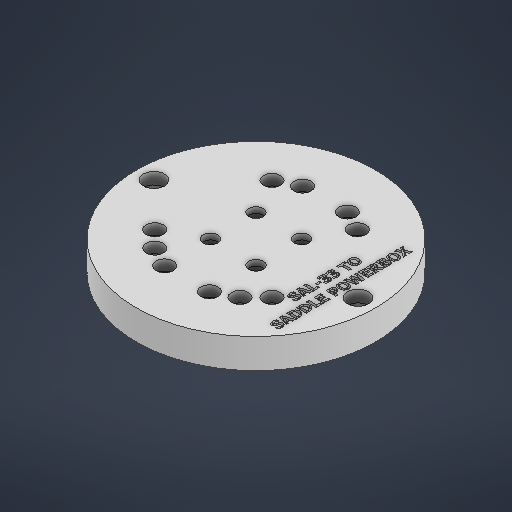
# Autodesk Inventor part: SAL-33 to Saddle Powerbox Adapter
Saved by Autodesk Inventor 2026.2 (Build 302298010, 298A)
## iProperties
Created: 2026-05-21
Part Number: SAL-33 to Saddle Powerbox Adapter
Material: Generic
Document SubType Name: Modeling
Designer: incep
Density: 1 g/cm^3
Appearance: Default
Author: incep
## iProperties of the stored document SAL-33 to Saddle Powerbox Adapter_3DPrint.ipt
Created: 2026-05-21
Part Number: SAL-33 to Saddle Powerbox Adapter_3DPrint
Material: Generic
Document SubType Name: Modeling
Designer: incep
Density: 1 g/cm^3
Appearance: Default
Author: incep
Autodesk Inventor part; units mm, degrees
ref_plane "YZ Plane" through (0, 0, 0) normal (1, 0, 0) x (0, 1, 0)
ref_plane "XZ Plane" through (0, 0, 0) normal (0, 1, 0) x (-1, 0, 0)
ref_plane "XY Plane" through (0, 0, 0) normal (0, 0, 1) x (1, 0, 0)
sketch "Sketch1" plane through (0, 0, 0) normal (0, 1, 0) x (-1, 0, 0)
  circle A0 centre (0, 0) radius 44.5
  circle A1 centre (0, 0) radius 22.75
  circle A2 centre (0, 0) radius 27 construction
  circle A3 centre (0, 27) radius 1.925 construction
  circle A4 centre (-8.3435, 25.6785) radius 1.925
  circle A5 centre (-15.8702, 21.8435) radius 1.925
  circle A6 centre (-21.8435, 15.8702) radius 1.925
  circle A7 centre (-25.6785, 8.3435) radius 1.925 construction
  circle A8 centre (-27, 0) radius 1.925 construction
  circle A9 centre (-25.6785, -8.3435) radius 1.925 construction
  circle A10 centre (-21.8435, -15.8702) radius 1.925 construction
  circle A11 centre (-15.8702, -21.8435) radius 1.925
  circle A12 centre (-8.3435, -25.6785) radius 1.925
  circle A13 centre (0, -27) radius 1.925 construction
  circle A14 centre (8.3435, -25.6785) radius 1.925
  circle A15 centre (15.8702, -21.8435) radius 1.925
  circle A16 centre (21.8435, -15.8702) radius 1.925 construction
  circle A17 centre (25.6785, -8.3435) radius 1.925 construction
  circle A18 centre (27, 0) radius 1.925 construction
  circle A19 centre (25.6785, 8.3435) radius 1.925 construction
  circle A20 centre (21.8435, 15.8702) radius 1.925
  circle A21 centre (15.8702, 21.8435) radius 1.925
  circle A22 centre (8.3435, 25.6785) radius 1.925
  dimension "d2" = 54
  dimension "d0" = 89
  dimension "d1" = 45.5
  dimension "d3" = 3.85
  dimension "d6" = 360
  constraints: 22 centre point, 3 coincident, 1 vertical alignment, 43 other
  measures "d0" diameter of A0
  measures "d1" diameter of A1
  measures "d3" diameter of A3
extrude "Extrusion1" add sketch "Sketch1" along normal blind 3
sketch "Sketch2" plane through (0, 3, 0) normal (0, 1, 0) x (1, 0, 0)
  circle A0 centre (0, 0) radius 22.75 projected
  circle A1 centre (0, 0) radius 44.5 projected
  circle A2 centre (-8.3435, -25.6785) radius 1.925 projected
  circle A3 centre (-15.8702, -21.8435) radius 1.925 projected
  circle A4 centre (-21.8435, -15.8702) radius 1.925 projected
  circle A5 centre (-15.8702, 21.8435) radius 1.925 projected
  circle A6 centre (-8.3435, 25.6785) radius 1.925 projected
  circle A7 centre (8.3435, 25.6785) radius 1.925 projected
  circle A8 centre (15.8702, 21.8435) radius 1.925 projected
  circle A9 centre (21.8435, -15.8702) radius 1.925 projected
  circle A10 centre (15.8702, -21.8435) radius 1.925 projected
  circle A11 centre (8.3435, -25.6785) radius 1.925 projected
  circle A12 centre (0, 0) radius 22.75 projected
extrude "Extrusion2" add sketch "Sketch2" along normal blind 8 contours A0 | A1
sketch "Sketch3" plane through (0, 11, 0) normal (0, 1, 0) x (1, 0, 0)
  circle A0 centre (0, 0) radius 44.5 projected
  circle A1 centre (0, 0) radius 44.5 projected
  circle A2 centre (8.3435, -25.6785) radius 1.925 projected
  circle A3 centre (15.8702, -21.8435) radius 1.925 projected
  circle A4 centre (21.8435, -15.8702) radius 1.925 projected
  circle A5 centre (15.8702, 21.8435) radius 1.925 projected
  circle A6 centre (8.3435, 25.6785) radius 1.925 projected
  circle A7 centre (-8.3435, 25.6785) radius 1.925 projected
  circle A8 centre (-15.8702, 21.8435) radius 1.925 projected
  circle A9 centre (-21.8435, -15.8702) radius 1.925 projected
  circle A10 centre (-15.8702, -21.8435) radius 1.925 projected
  circle A11 centre (-8.3435, -25.6785) radius 1.925 projected
  circle A12 centre (-8.3435, -25.6785) radius 3.2
  circle A13 centre (-21.8435, -15.8702) radius 3.2
  circle A14 centre (-15.8702, -21.8435) radius 3.2
  circle A15 centre (8.3435, -25.6785) radius 3.2
  circle A16 centre (15.8702, -21.8435) radius 3.2
  circle A17 centre (21.8435, -15.8702) radius 3.2
  circle A18 centre (15.8702, 21.8435) radius 3.2
  circle A19 centre (8.3435, 25.6785) radius 3.2
  circle A20 centre (-8.3435, 25.6785) radius 3.2
  circle A21 centre (-15.8702, 21.8435) radius 3.2
  dimension "d12" = 6.4
  dimension "d13" = 6.4
  dimension "d14" = 6.4
  dimension "d15" = 6.4
  dimension "d16" = 6.4
  dimension "d17" = 6.4
  dimension "d18" = 6.4
  dimension "d19" = 6.4
  dimension "d20" = 6.4
  dimension "d21" = 6.4
  constraints: 10 centre point, 10 coincident
  measures "d12" diameter of A12
  measures "d13" diameter of A13
  measures "d14" diameter of A14
  measures "d15" diameter of A15
  measures "d16" diameter of A16
  measures "d17" diameter of A17
  measures "d18" diameter of A18
  measures "d19" diameter of A19
  measures "d20" diameter of A20
  measures "d21" diameter of A21
extrude "Extrusion3" cut sketch "Sketch3" against normal blind 4 contours A2 | A3 | A4 | A5 | A6 | A7 | A8 | A9 | A10 | A11 | A12 | A13 | A14 | A15 | A16 | A17 | A18 | A19 | A20 | A21
sketch "Sketch4" plane through (0, 11, 0) normal (0, 1, 0) x (1, 0, 0)
  circle A0 centre (-38, 0) radius 3.925
  circle A1 centre (38, 0) radius 3.925
  line L0 (-38, 0) -> (38, 0) construction
  circle A2 centre (-38, 0) radius 2.25
  circle A3 centre (38, 0) radius 2.25
  point P0 (0, 0)
  point P1 (0, 0)
  dimension "d24" = 7.85
  dimension "d25" = 76
  dimension "d26" = 4.5
  constraints: 4 centre point, 3 coincident, 2 end point, 2 equal radius, 2 horizontal alignment, 1 horizontal, 1 midpoint
  measures "d24" diameter of A0
  measures "d25" distance of L0.end L0.start
  measures "d26" diameter of A2
extrude "Extrusion4" cut sketch "Sketch4" against normal blind 4.36 contours A0 | A1 | A2 | A3
extrude "Extrusion5" cut sketch "Sketch4" against normal up to surface (11 mm away) contours A2 | A3
sketch "Sketch5" plane through (0, 11, 0) normal (0, 1, 0) x (1, 0, 0)
  line L0 (-8.5, -8.5) -> (8.5, -8.5) construction
  line L1 (8.5, -8.5) -> (8.5, 8.5) construction
  line L2 (8.5, 8.5) -> (-8.5, 8.5) construction
  line L3 (-8.5, 8.5) -> (-8.5, -8.5) construction
  circle A0 centre (-8.5, -8.5) radius 2.7
  circle A1 centre (-8.5, 8.5) radius 2.7
  circle A2 centre (8.5, 8.5) radius 2.7
  circle A3 centre (8.5, -8.5) radius 2.7
  circle A4 centre (0, 0) radius 12.0208 construction
  point P0 (-8.5, 0)
  point P1 (0, 8.5)
  dimension "d40" = 24.0416
  dimension "d31" = 5.4
  dimension "d37" = 17
  constraints: 8 end point, 5 coincident, 4 centre point, 3 equal radius, 2 midpoint, 2 parallel, 2 perpendicular, 1 horizontal, 1 horizontal alignment, 1 vertical alignment, 3 other
  measures "d31" diameter of A0
  measures "d37" distance of L0.start L0.end
extrude "Extrusion6" cut sketch "Sketch5" against normal up to surface (8 mm away)
sketch "Sketch6" plane through (0, 3, 0) normal (0, -1, 0) x (1, 0, 0)
  circle A0 centre (8.5, -8.5) radius 2.7 projected
  circle A1 centre (-8.5, 8.5) radius 2.7 projected
  circle A2 centre (-8.5, -8.5) radius 2.7 projected
  circle A3 centre (8.5, 8.5) radius 2.7 projected
  circle A4 centre (0, 0) radius 22.75 projected
  circle A5 centre (-8.5, 8.5) radius 3.2
  circle A6 centre (8.5, 8.5) radius 3.2
  circle A7 centre (-8.5, -8.5) radius 3.2
  circle A8 centre (8.5, -8.5) radius 3.2
  dimension "d34" = 6.4
  constraints: 4 centre point, 4 coincident, 3 equal radius
  measures "d34" diameter of A5
extrude "Extrusion7" cut sketch "Sketch6" against normal blind 5.8 contours A0 | A1 | A2 | A3 | A5 | A6 | A7 | A8
sketch "Sketch7" plane through (0, 11, 0) normal (0, 1, 0) x (1, 0, 0)
  line L0 (23.7791, -32.5352) -> (23.7791, 32.5352) construction
  line L1 (23.7791, 32.5352) -> (26.5195, 32.5352) construction
  line L2 (26.5195, 32.5352) -> (26.5195, -32.5352) construction
  line L3 (26.5195, -32.5352) -> (23.7791, -32.5352) construction
  spline S0 degree 2 poles (27.4734, -11.4216) (27.4734, -11.8308) (27.3149, -12.4474) (27.1997, -12.7126) knots 0 0 0 1 2 2 2
  line L4 (27.1997, -12.7126) -> (26.3525, -12.7126)
  line L5 (26.3525, -12.7126) -> (26.3525, -12.6319)
  spline S1 degree 2 poles (26.3525, -12.6319) (26.5801, -12.3639) (26.825, -11.7213) (26.825, -11.4187) knots 0 0 0 1 2 2 2
  spline S2 degree 2 poles (26.825, -11.4187) (26.825, -11.3409) (26.7905, -11.0902) (26.7559, -11.0152) knots 0 0 0 1 2 2 2
  spline S3 degree 2 poles (26.7559, -11.0152) (26.7155, -10.923) (26.5686, -10.7934) (26.4504, -10.7934) knots 0 0 0 1 2 2 2
  spline S4 degree 2 poles (26.4504, -10.7934) (26.315, -10.7934) (26.1479, -11.0037) (26.1104, -11.1478) knots 0 0 0 1 2 2 2
  spline S5 degree 2 poles (26.1104, -11.1478) (26.0614, -11.3293) (25.9778, -11.7414) (25.9144, -11.923) knots 0 0 0 1 2 2 2
  spline S6 degree 2 poles (25.9144, -11.923) (25.7704, -12.3351) (25.2776, -12.6924) (24.9087, -12.6924) knots 0 0 0 1 2 2 2
  spline S7 degree 2 poles (24.9087, -12.6924) (24.4102, -12.6924) (23.7906, -11.8481) (23.7906, -11.2141) knots 0 0 0 1 2 2 2
  spline S8 degree 2 poles (23.7906, -11.2141) (23.7906, -10.8971) (23.9203, -10.2689) (24.0298, -10.0211) knots 0 0 0 1 2 2 2
  line L6 (24.0298, -10.0211) -> (24.8424, -10.0211)
  line L7 (24.8424, -10.0211) -> (24.8424, -10.0989)
  spline S9 degree 2 poles (24.8424, -10.0989) (24.6724, -10.2977) (24.439, -10.8683) (24.439, -11.168) knots 0 0 0 1 2 2 2
  spline S10 degree 2 poles (24.439, -11.168) (24.439, -11.2861) (24.4736, -11.4705) (24.5197, -11.5743) knots 0 0 0 1 2 2 2
  spline S11 degree 2 poles (24.5197, -11.5743) (24.5572, -11.6579) (24.707, -11.7789) (24.7992, -11.7789) knots 0 0 0 1 2 2 2
  spline S12 degree 2 poles (24.7992, -11.7789) (24.9375, -11.7789) (25.096, -11.5858) (25.1594, -11.3092) knots 0 0 0 1 2 2 2
  spline S13 degree 2 poles (25.1594, -11.3092) (25.1998, -11.1305) (25.2776, -10.7991) (25.3439, -10.6089) knots 0 0 0 1 2 2 2
  spline S14 degree 2 poles (25.3439, -10.6089) (25.4793, -10.2401) (25.9288, -9.8799) (26.2977, -9.8799) knots 0 0 0 1 2 2 2
  spline S15 degree 2 poles (26.2977, -9.8799) (26.8279, -9.8799) (27.4734, -10.7127) (27.4734, -11.4216) knots 0 0 0 1 2 2 2
  line L8 (27.41, -9.8049) -> (23.854, -8.6033)
  line L9 (23.854, -8.6033) -> (23.854, -7.6293)
  line L10 (23.854, -7.6293) -> (27.41, -6.4276)
  line L11 (27.41, -6.4276) -> (27.41, -7.3469)
  line L12 (27.41, -7.3469) -> (26.6838, -7.5687)
  line L13 (26.6838, -7.5687) -> (26.6838, -8.6868)
  line L14 (26.6838, -8.6868) -> (27.41, -8.9116)
  line L15 (27.41, -8.9116) -> (27.41, -9.8049)
  line L16 (26.0383, -7.7647) -> (24.8626, -8.1278)
  line L17 (24.8626, -8.1278) -> (26.0383, -8.4938)
  line L18 (26.0383, -8.4938) -> (26.0383, -7.7647)
  line L19 (27.41, -3.7015) -> (27.41, -6.0732)
  line L20 (27.41, -6.0732) -> (23.854, -6.0732)
  line L21 (23.854, -6.0732) -> (23.854, -5.1798)
  line L22 (23.854, -5.1798) -> (26.7328, -5.1798)
  line L23 (26.7328, -5.1798) -> (26.7328, -3.7015)
  line L24 (26.7328, -3.7015) -> (27.41, -3.7015)
  line L25 (26.1709, -1.7996) -> (26.1709, -3.3817)
  line L26 (26.1709, -3.3817) -> (25.5081, -3.3817)
  line L27 (25.5081, -3.3817) -> (25.5081, -1.7996)
  line L28 (25.5081, -1.7996) -> (26.1709, -1.7996)
  spline S16 degree 2 poles (26.3323, 1.3501) (26.5945, 1.3501) (27.0239, 1.157) (27.1737, 0.9697) knots 0 0 0 1 2 2 2
  spline S17 degree 2 poles (27.1737, 0.9697) (27.3236, 0.7824) (27.485, 0.2723) (27.485, -0.0937) knots 0 0 0 1 2 2 2
  spline S18 degree 2 poles (27.485, -0.0937) (27.485, -0.5086) (27.3466, -1.1022) (27.2602, -1.2896) knots 0 0 0 1 2 2 2
  line L29 (27.2602, -1.2896) -> (26.4879, -1.2896)
  line L30 (26.4879, -1.2896) -> (26.4879, -1.2031)
  spline S19 degree 2 poles (26.4879, -1.2031) (26.6118, -1.0071) (26.7962, -0.4798) (26.7962, -0.2608) knots 0 0 0 1 2 2 2
  spline S20 degree 2 poles (26.7962, -0.2608) (26.7962, -0.1311) (26.7501, 0.1715) (26.6752, 0.2752) knots 0 0 0 1 2 2 2
  spline S21 degree 2 poles (26.6752, 0.2752) (26.6147, 0.3559) (26.4389, 0.4539) (26.2804, 0.4539) knots 0 0 0 1 2 2 2
  spline S22 degree 2 poles (26.2804, 0.4539) (26.1219, 0.4539) (25.9519, 0.3155) (25.9116, 0.2003) knots 0 0 0 1 2 2 2
  spline S23 degree 2 poles (25.9116, 0.2003) (25.8712, 0.085) (25.8626, -0.2349) (25.8626, -0.3588) knots 0 0 0 1 2 2 2
  line L31 (25.8626, -0.3588) -> (25.8626, -0.5115)
  line L32 (25.8626, -0.5115) -> (25.2372, -0.5115)
  line L33 (25.2372, -0.5115) -> (25.2372, -0.3703)
  spline S24 degree 2 poles (25.2372, -0.3703) (25.2372, -0.2089) (25.2084, 0.0648) (25.1652, 0.1599) knots 0 0 0 1 2 2 2
  spline S25 degree 2 poles (25.1652, 0.1599) (25.1191, 0.255) (24.9577, 0.3617) (24.8194, 0.3617) knots 0 0 0 1 2 2 2
  spline S26 degree 2 poles (24.8194, 0.3617) (24.7099, 0.3617) (24.5745, 0.2608) (24.537, 0.1888) knots 0 0 0 1 2 2 2
  spline S27 degree 2 poles (24.537, 0.1888) (24.4938, 0.1023) (24.4649, -0.1282) (24.4649, -0.2089) knots 0 0 0 1 2 2 2
  spline S28 degree 2 poles (24.4649, -0.2089) (24.4649, -0.3386) (24.5255, -0.6124) (24.5745, -0.7392) knots 0 0 0 1 2 2 2
  spline S29 degree 2 poles (24.5745, -0.7392) (24.6119, -0.84) (24.7329, -1.059) (24.7646, -1.1109) knots 0 0 0 1 2 2 2
  line L34 (24.7646, -1.1109) -> (24.7646, -1.1858)
  line L35 (24.7646, -1.1858) -> (24.0039, -1.1858)
  spline S30 degree 2 poles (24.0039, -1.1858) (23.9261, -1.0014) (23.7791, -0.3789) (23.7791, -0.0533) knots 0 0 0 1 2 2 2
  spline S31 degree 2 poles (23.7791, -0.0533) (23.7791, 0.2637) (23.8886, 0.7305) (23.9952, 0.8948) knots 0 0 0 1 2 2 2
  spline S32 degree 2 poles (23.9952, 0.8948) (24.1076, 1.0763) (24.4534, 1.2579) (24.6695, 1.2579) knots 0 0 0 1 2 2 2
  spline S33 degree 2 poles (24.6695, 1.2579) (24.975, 1.2579) (25.4303, 0.9063) (25.4966, 0.6181) knots 0 0 0 1 2 2 2
  line L36 (25.4966, 0.6181) -> (25.5312, 0.6181)
  spline S34 degree 2 poles (25.5312, 0.6181) (25.5485, 0.7449) (25.6407, 0.987) (25.7444, 1.1022) knots 0 0 0 1 2 2 2
  spline S35 degree 2 poles (25.7444, 1.1022) (25.8366, 1.2089) (26.1306, 1.3501) (26.3323, 1.3501) knots 0 0 0 1 2 2 2
  spline S36 degree 2 poles (26.3323, 4.4652) (26.5945, 4.4652) (27.0239, 4.2721) (27.1737, 4.0848) knots 0 0 0 1 2 2 2
  spline S37 degree 2 poles (27.1737, 4.0848) (27.3236, 3.8975) (27.485, 3.3874) (27.485, 3.0214) knots 0 0 0 1 2 2 2
  spline S38 degree 2 poles (27.485, 3.0214) (27.485, 2.6065) (27.3466, 2.0129) (27.2602, 1.8255) knots 0 0 0 1 2 2 2
  line L37 (27.2602, 1.8255) -> (26.4879, 1.8255)
  line L38 (26.4879, 1.8255) -> (26.4879, 1.912)
  spline S39 degree 2 poles (26.4879, 1.912) (26.6118, 2.108) (26.7962, 2.6353) (26.7962, 2.8543) knots 0 0 0 1 2 2 2
  spline S40 degree 2 poles (26.7962, 2.8543) (26.7962, 2.984) (26.7501, 3.2866) (26.6752, 3.3903) knots 0 0 0 1 2 2 2
  spline S41 degree 2 poles (26.6752, 3.3903) (26.6147, 3.471) (26.4389, 3.569) (26.2804, 3.569) knots 0 0 0 1 2 2 2
  spline S42 degree 2 poles (26.2804, 3.569) (26.1219, 3.569) (25.9519, 3.4306) (25.9116, 3.3154) knots 0 0 0 1 2 2 2
  spline S43 degree 2 poles (25.9116, 3.3154) (25.8712, 3.2001) (25.8626, 2.8802) (25.8626, 2.7563) knots 0 0 0 1 2 2 2
  line L39 (25.8626, 2.7563) -> (25.8626, 2.6036)
  line L40 (25.8626, 2.6036) -> (25.2372, 2.6036)
  line L41 (25.2372, 2.6036) -> (25.2372, 2.7448)
  spline S44 degree 2 poles (25.2372, 2.7448) (25.2372, 2.9062) (25.2084, 3.1799) (25.1652, 3.275) knots 0 0 0 1 2 2 2
  spline S45 degree 2 poles (25.1652, 3.275) (25.1191, 3.3701) (24.9577, 3.4768) (24.8194, 3.4768) knots 0 0 0 1 2 2 2
  spline S46 degree 2 poles (24.8194, 3.4768) (24.7099, 3.4768) (24.5745, 3.3759) (24.537, 3.3039) knots 0 0 0 1 2 2 2
  spline S47 degree 2 poles (24.537, 3.3039) (24.4938, 3.2174) (24.4649, 2.9869) (24.4649, 2.9062) knots 0 0 0 1 2 2 2
  spline S48 degree 2 poles (24.4649, 2.9062) (24.4649, 2.7765) (24.5255, 2.5027) (24.5745, 2.3759) knots 0 0 0 1 2 2 2
  spline S49 degree 2 poles (24.5745, 2.3759) (24.6119, 2.2751) (24.7329, 2.0561) (24.7646, 2.0042) knots 0 0 0 1 2 2 2
  line L42 (24.7646, 2.0042) -> (24.7646, 1.9293)
  line L43 (24.7646, 1.9293) -> (24.0039, 1.9293)
  spline S50 degree 2 poles (24.0039, 1.9293) (23.9261, 2.1137) (23.7791, 2.7362) (23.7791, 3.0618) knots 0 0 0 1 2 2 2
  spline S51 degree 2 poles (23.7791, 3.0618) (23.7791, 3.3788) (23.8886, 3.8456) (23.9952, 4.0099) knots 0 0 0 1 2 2 2
  spline S52 degree 2 poles (23.9952, 4.0099) (24.1076, 4.1914) (24.4534, 4.373) (24.6695, 4.373) knots 0 0 0 1 2 2 2
  spline S53 degree 2 poles (24.6695, 4.373) (24.975, 4.373) (25.4303, 4.0214) (25.4966, 3.7332) knots 0 0 0 1 2 2 2
  line L44 (25.4966, 3.7332) -> (25.5312, 3.7332)
  spline S54 degree 2 poles (25.5312, 3.7332) (25.5485, 3.86) (25.6407, 4.1021) (25.7444, 4.2173) knots 0 0 0 1 2 2 2
  spline S55 degree 2 poles (25.7444, 4.2173) (25.8366, 4.324) (26.1306, 4.4652) (26.3323, 4.4652) knots 0 0 0 1 2 2 2
  line L45 (27.41, 7.1797) -> (24.5312, 7.1797)
  line L46 (24.5312, 7.1797) -> (24.5312, 6.1279)
  line L47 (24.5312, 6.1279) -> (23.854, 6.1279)
  line L48 (23.854, 6.1279) -> (23.854, 9.1249)
  line L49 (23.854, 9.1249) -> (24.5312, 9.1249)
  line L50 (24.5312, 9.1249) -> (24.5312, 8.073)
  line L51 (24.5312, 8.073) -> (27.41, 8.073)
  line L52 (27.41, 8.073) -> (27.41, 7.1797)
  spline S56 degree 2 poles (25.632, 12.727) (26.4965, 12.727) (27.485, 11.8048) (27.485, 11.0037) knots 0 0 0 1 2 2 2
  spline S57 degree 2 poles (27.485, 11.0037) (27.485, 10.1997) (26.485, 9.2834) (25.632, 9.2834) knots 0 0 0 1 2 2 2
  spline S58 degree 2 poles (25.632, 9.2834) (24.7762, 9.2834) (23.7791, 10.1997) (23.7791, 11.0037) knots 0 0 0 1 2 2 2
  spline S59 degree 2 poles (23.7791, 11.0037) (23.7791, 11.8048) (24.7704, 12.727) (25.632, 12.727) knots 0 0 0 1 2 2 2
  spline S60 degree 2 poles (25.632, 11.8048) (25.3122, 11.8048) (24.8655, 11.6751) (24.7243, 11.5628) knots 0 0 0 1 2 2 2
  spline S61 degree 2 poles (24.7243, 11.5628) (24.5773, 11.4504) (24.4505, 11.1622) (24.4505, 11.0066) knots 0 0 0 1 2 2 2
  spline S62 degree 2 poles (24.4505, 11.0066) (24.4505, 10.8423) (24.5687, 10.5743) (24.7185, 10.4504) knots 0 0 0 1 2 2 2
  spline S63 degree 2 poles (24.7185, 10.4504) (24.8569, 10.3409) (25.315, 10.2055) (25.632, 10.2055) knots 0 0 0 1 2 2 2
  spline S64 degree 2 poles (25.632, 10.2055) (25.9605, 10.2055) (26.3928, 10.3352) (26.5398, 10.4476) knots 0 0 0 1 2 2 2
  spline S65 degree 2 poles (26.5398, 10.4476) (26.6867, 10.5599) (26.8135, 10.851) (26.8135, 11.0066) knots 0 0 0 1 2 2 2
  spline S66 degree 2 poles (26.8135, 11.0066) (26.8135, 11.1651) (26.6781, 11.459) (26.534, 11.5656) knots 0 0 0 1 2 2 2
  spline S67 degree 2 poles (26.534, 11.5656) (26.3784, 11.6809) (25.9663, 11.8048) (25.632, 11.8048) knots 0 0 0 1 2 2 2
  spline S68 degree 2 poles (33.3283, -23.6241) (33.3283, -24.0333) (33.1698, -24.6499) (33.0545, -24.9151) knots 0 0 0 1 2 2 2
  line L53 (33.0545, -24.9151) -> (32.2073, -24.9151)
  line L54 (32.2073, -24.9151) -> (32.2073, -24.8344)
  spline S69 degree 2 poles (32.2073, -24.8344) (32.435, -24.5664) (32.6799, -23.9238) (32.6799, -23.6212) knots 0 0 0 1 2 2 2
  spline S70 degree 2 poles (32.6799, -23.6212) (32.6799, -23.5434) (32.6453, -23.2927) (32.6107, -23.2177) knots 0 0 0 1 2 2 2
  spline S71 degree 2 poles (32.6107, -23.2177) (32.5704, -23.1255) (32.4234, -22.9958) (32.3053, -22.9958) knots 0 0 0 1 2 2 2
  spline S72 degree 2 poles (32.3053, -22.9958) (32.1699, -22.9958) (32.0027, -23.2062) (31.9653, -23.3503) knots 0 0 0 1 2 2 2
  spline S73 degree 2 poles (31.9653, -23.3503) (31.9163, -23.5318) (31.8327, -23.9439) (31.7693, -24.1255) knots 0 0 0 1 2 2 2
  spline S74 degree 2 poles (31.7693, -24.1255) (31.6252, -24.5376) (31.1324, -24.8949) (30.7636, -24.8949) knots 0 0 0 1 2 2 2
  spline S75 degree 2 poles (30.7636, -24.8949) (30.2651, -24.8949) (29.6455, -24.0505) (29.6455, -23.4166) knots 0 0 0 1 2 2 2
  spline S76 degree 2 poles (29.6455, -23.4166) (29.6455, -23.0996) (29.7752, -22.4714) (29.8847, -22.2236) knots 0 0 0 1 2 2 2
  line L55 (29.8847, -22.2236) -> (30.6973, -22.2236)
  line L56 (30.6973, -22.2236) -> (30.6973, -22.3014)
  spline S77 degree 2 poles (30.6973, -22.3014) (30.5273, -22.5002) (30.2939, -23.0708) (30.2939, -23.3705) knots 0 0 0 1 2 2 2
  spline S78 degree 2 poles (30.2939, -23.3705) (30.2939, -23.4886) (30.3285, -23.673) (30.3746, -23.7768) knots 0 0 0 1 2 2 2
  spline S79 degree 2 poles (30.3746, -23.7768) (30.412, -23.8604) (30.5619, -23.9814) (30.6541, -23.9814) knots 0 0 0 1 2 2 2
  spline S80 degree 2 poles (30.6541, -23.9814) (30.7924, -23.9814) (30.9509, -23.7883) (31.0143, -23.5117) knots 0 0 0 1 2 2 2
  spline S81 degree 2 poles (31.0143, -23.5117) (31.0546, -23.333) (31.1324, -23.0016) (31.1987, -22.8114) knots 0 0 0 1 2 2 2
  spline S82 degree 2 poles (31.1987, -22.8114) (31.3342, -22.4426) (31.7837, -22.0824) (32.1526, -22.0824) knots 0 0 0 1 2 2 2
  spline S83 degree 2 poles (32.1526, -22.0824) (32.6828, -22.0824) (33.3283, -22.9152) (33.3283, -23.6241) knots 0 0 0 1 2 2 2
  line L57 (33.2649, -22.0074) -> (29.7089, -20.8058)
  line L58 (29.7089, -20.8058) -> (29.7089, -19.8318)
  line L59 (29.7089, -19.8318) -> (33.2649, -18.6301)
  line L60 (33.2649, -18.6301) -> (33.2649, -19.5494)
  line L61 (33.2649, -19.5494) -> (32.5387, -19.7712)
  line L62 (32.5387, -19.7712) -> (32.5387, -20.8893)
  line L63 (32.5387, -20.8893) -> (33.2649, -21.1141)
  line L64 (33.2649, -21.1141) -> (33.2649, -22.0074)
  line L65 (31.8932, -19.9672) -> (30.7175, -20.3303)
  line L66 (30.7175, -20.3303) -> (31.8932, -20.6963)
  line L67 (31.8932, -20.6963) -> (31.8932, -19.9672)
  spline S84 degree 2 poles (31.4898, -15.1029) (31.9883, -15.1029) (32.7721, -15.538) (32.9825, -15.8694) knots 0 0 0 1 2 2 2
  spline S85 degree 2 poles (32.9825, -15.8694) (33.1612, -16.1461) (33.2649, -16.7973) (33.2649, -17.1633) knots 0 0 0 1 2 2 2
  line L68 (33.2649, -17.1633) -> (33.2649, -18.2756)
  line L69 (33.2649, -18.2756) -> (29.7089, -18.2756)
  line L70 (29.7089, -18.2756) -> (29.7089, -17.1748)
  spline S86 degree 2 poles (29.7089, -17.1748) (29.7089, -16.8002) (29.804, -16.1461) (29.9884, -15.8579) knots 0 0 0 1 2 2 2
  spline S87 degree 2 poles (29.9884, -15.8579) (30.2132, -15.5092) (30.974, -15.1029) (31.4898, -15.1029) knots 0 0 0 1 2 2 2
  spline S88 degree 2 poles (31.484, -16.0193) (31.1324, -16.0193) (30.631, -16.2614) (30.4898, -16.5092) knots 0 0 0 1 2 2 2
  spline S89 degree 2 poles (30.4898, -16.5092) (30.3919, -16.6907) (30.3717, -17.0884) (30.3717, -17.365) knots 0 0 0 1 2 2 2
  line L71 (30.3717, -17.365) -> (30.3717, -17.3823)
  line L72 (30.3717, -17.3823) -> (32.5992, -17.3823)
  line L73 (32.5992, -17.3823) -> (32.5992, -17.365)
  spline S90 degree 2 poles (32.5992, -17.365) (32.5992, -17.0653) (32.5791, -16.6533) (32.4609, -16.466) knots 0 0 0 1 2 2 2
  spline S91 degree 2 poles (32.4609, -16.466) (32.3226, -16.2469) (31.8356, -16.0193) (31.484, -16.0193) knots 0 0 0 1 2 2 2
  spline S92 degree 2 poles (31.4898, -11.3999) (31.9883, -11.3999) (32.7721, -11.8351) (32.9825, -12.1665) knots 0 0 0 1 2 2 2
  spline S93 degree 2 poles (32.9825, -12.1665) (33.1612, -12.4431) (33.2649, -13.0944) (33.2649, -13.4604) knots 0 0 0 1 2 2 2
  line L74 (33.2649, -13.4604) -> (33.2649, -14.5727)
  line L75 (33.2649, -14.5727) -> (29.7089, -14.5727)
  line L76 (29.7089, -14.5727) -> (29.7089, -13.4719)
  spline S94 degree 2 poles (29.7089, -13.4719) (29.7089, -13.0973) (29.804, -12.4431) (29.9884, -12.1549) knots 0 0 0 1 2 2 2
  spline S95 degree 2 poles (29.9884, -12.1549) (30.2132, -11.8063) (30.974, -11.3999) (31.4898, -11.3999) knots 0 0 0 1 2 2 2
  spline S96 degree 2 poles (31.484, -12.3163) (31.1324, -12.3163) (30.631, -12.5584) (30.4898, -12.8062) knots 0 0 0 1 2 2 2
  spline S97 degree 2 poles (30.4898, -12.8062) (30.3919, -12.9878) (30.3717, -13.3854) (30.3717, -13.6621) knots 0 0 0 1 2 2 2
  line L77 (30.3717, -13.6621) -> (30.3717, -13.6794)
  line L78 (30.3717, -13.6794) -> (32.5992, -13.6794)
  line L79 (32.5992, -13.6794) -> (32.5992, -13.6621)
  spline S98 degree 2 poles (32.5992, -13.6621) (32.5992, -13.3624) (32.5791, -12.9503) (32.4609, -12.763) knots 0 0 0 1 2 2 2
  spline S99 degree 2 poles (32.4609, -12.763) (32.3226, -12.544) (31.8356, -12.3163) (31.484, -12.3163) knots 0 0 0 1 2 2 2
  line L80 (33.2649, -8.4981) -> (33.2649, -10.8697)
  line L81 (33.2649, -10.8697) -> (29.7089, -10.8697)
  line L82 (29.7089, -10.8697) -> (29.7089, -9.9764)
  line L83 (29.7089, -9.9764) -> (32.5877, -9.9764)
  line L84 (32.5877, -9.9764) -> (32.5877, -8.4981)
  line L85 (32.5877, -8.4981) -> (33.2649, -8.4981)
  line L86 (33.2649, -8.0716) -> (29.7089, -8.0716)
  line L87 (29.7089, -8.0716) -> (29.7089, -5.6683)
  line L88 (29.7089, -5.6683) -> (30.3861, -5.6683)
  line L89 (30.3861, -5.6683) -> (30.3861, -7.184)
  line L90 (30.3861, -7.184) -> (31.0114, -7.184)
  line L91 (31.0114, -7.184) -> (31.0114, -5.7864)
  line L92 (31.0114, -5.7864) -> (31.6886, -5.7864)
  line L93 (31.6886, -5.7864) -> (31.6886, -7.184)
  line L94 (31.6886, -7.184) -> (32.5877, -7.184)
  line L95 (32.5877, -7.184) -> (32.5877, -5.6683)
  line L96 (32.5877, -5.6683) -> (33.2649, -5.6683)
  line L97 (33.2649, -5.6683) -> (33.2649, -8.0716)
  spline S100 degree 2 poles (30.8299, -0.8962) (31.0777, -0.8962) (31.5272, -1.0547) (31.6771, -1.2017) knots 0 0 0 1 2 2 2
  spline S101 degree 2 poles (31.6771, -1.2017) (31.7722, -1.291) (31.9278, -1.51) (31.9825, -1.6397) knots 0 0 0 1 2 2 2
  spline S102 degree 2 poles (31.9825, -1.6397) (32.0373, -1.7722) (32.1007, -2.0806) (32.1007, -2.2708) knots 0 0 0 1 2 2 2
  line L98 (32.1007, -2.2708) -> (32.1007, -2.7376)
  line L99 (32.1007, -2.7376) -> (33.2649, -2.7376)
  line L100 (33.2649, -2.7376) -> (33.2649, -3.6309)
  line L101 (33.2649, -3.6309) -> (29.7089, -3.6309)
  line L102 (29.7089, -3.6309) -> (29.7089, -2.2506)
  spline S103 degree 2 poles (29.7089, -2.2506) (29.7089, -1.9451) (29.8213, -1.4985) (29.9423, -1.3169) knots 0 0 0 1 2 2 2
  spline S104 degree 2 poles (29.9423, -1.3169) (30.0777, -1.1152) (30.5215, -0.8962) (30.8299, -0.8962) knots 0 0 0 1 2 2 2
  spline S105 degree 2 poles (30.8529, -1.8126) (30.7002, -1.8126) (30.4841, -1.9567) (30.4437, -2.0546) knots 0 0 0 1 2 2 2
  spline S106 degree 2 poles (30.4437, -2.0546) (30.389, -2.1814) (30.3717, -2.412) (30.3717, -2.6108) knots 0 0 0 1 2 2 2
  line L103 (30.3717, -2.6108) -> (30.3717, -2.7376)
  line L104 (30.3717, -2.7376) -> (31.4379, -2.7376)
  line L105 (31.4379, -2.7376) -> (31.4379, -2.6742)
  spline S107 degree 2 poles (31.4379, -2.6742) (31.4379, -2.5503) (31.4321, -2.3255) (31.4177, -2.242) knots 0 0 0 1 2 2 2
  spline S108 degree 2 poles (31.4177, -2.242) (31.4062, -2.1699) (31.337, -2.0114) (31.2938, -1.9682) knots 0 0 0 1 2 2 2
  spline S109 degree 2 poles (31.2938, -1.9682) (31.2074, -1.876) (31.0143, -1.8126) (30.8529, -1.8126) knots 0 0 0 1 2 2 2
  spline S110 degree 2 poles (31.4869, 2.8183) (32.3514, 2.8183) (33.3398, 1.8962) (33.3398, 1.095) knots 0 0 0 1 2 2 2
  spline S111 degree 2 poles (33.3398, 1.095) (33.3398, 0.2911) (32.3399, -0.6253) (31.4869, -0.6253) knots 0 0 0 1 2 2 2
  spline S112 degree 2 poles (31.4869, -0.6253) (30.631, -0.6253) (29.634, 0.2911) (29.634, 1.095) knots 0 0 0 1 2 2 2
  spline S113 degree 2 poles (29.634, 1.095) (29.634, 1.8962) (30.6253, 2.8183) (31.4869, 2.8183) knots 0 0 0 1 2 2 2
  spline S114 degree 2 poles (31.4869, 1.8962) (31.167, 1.8962) (30.7204, 1.7665) (30.5792, 1.6541) knots 0 0 0 1 2 2 2
  spline S115 degree 2 poles (30.5792, 1.6541) (30.4322, 1.5417) (30.3054, 1.2535) (30.3054, 1.0979) knots 0 0 0 1 2 2 2
  spline S116 degree 2 poles (30.3054, 1.0979) (30.3054, 0.9337) (30.4235, 0.6657) (30.5734, 0.5418) knots 0 0 0 1 2 2 2
  spline S117 degree 2 poles (30.5734, 0.5418) (30.7117, 0.4323) (31.1699, 0.2968) (31.4869, 0.2968) knots 0 0 0 1 2 2 2
  spline S118 degree 2 poles (31.4869, 0.2968) (31.8154, 0.2968) (32.2477, 0.4265) (32.3946, 0.5389) knots 0 0 0 1 2 2 2
  spline S119 degree 2 poles (32.3946, 0.5389) (32.5416, 0.6513) (32.6684, 0.9423) (32.6684, 1.0979) knots 0 0 0 1 2 2 2
  spline S120 degree 2 poles (32.6684, 1.0979) (32.6684, 1.2564) (32.5329, 1.5503) (32.3889, 1.657) knots 0 0 0 1 2 2 2
  spline S121 degree 2 poles (32.3889, 1.657) (32.2332, 1.7722) (31.8212, 1.8962) (31.4869, 1.8962) knots 0 0 0 1 2 2 2
  line L106 (29.7089, 7.9333) -> (33.2649, 7.0342)
  line L107 (33.2649, 7.0342) -> (33.2649, 6.0544)
  line L108 (33.2649, 6.0544) -> (31.0662, 5.4838)
  line L109 (31.0662, 5.4838) -> (33.2649, 4.9334)
  line L110 (33.2649, 4.9334) -> (33.2649, 3.9508)
  line L111 (33.2649, 3.9508) -> (29.7089, 3.0517)
  line L112 (29.7089, 3.0517) -> (29.7089, 3.9796)
  line L113 (29.7089, 3.9796) -> (32.0892, 4.4695)
  line L114 (32.0892, 4.4695) -> (29.7089, 5.0631)
  line L115 (29.7089, 5.0631) -> (29.7089, 5.9507)
  line L116 (29.7089, 5.9507) -> (32.092, 6.5155)
  line L117 (32.092, 6.5155) -> (29.7089, 7.0284)
  line L118 (29.7089, 7.0284) -> (29.7089, 7.9333)
  line L119 (33.2649, 8.3742) -> (29.7089, 8.3742)
  line L120 (29.7089, 8.3742) -> (29.7089, 10.7775)
  line L121 (29.7089, 10.7775) -> (30.3861, 10.7775)
  line L122 (30.3861, 10.7775) -> (30.3861, 9.2617)
  line L123 (30.3861, 9.2617) -> (31.0114, 9.2617)
  line L124 (31.0114, 9.2617) -> (31.0114, 10.6594)
  line L125 (31.0114, 10.6594) -> (31.6886, 10.6594)
  line L126 (31.6886, 10.6594) -> (31.6886, 9.2617)
  line L127 (31.6886, 9.2617) -> (32.5877, 9.2617)
  line L128 (32.5877, 9.2617) -> (32.5877, 10.7775)
  line L129 (32.5877, 10.7775) -> (33.2649, 10.7775)
  line L130 (33.2649, 10.7775) -> (33.2649, 8.3742)
  line L131 (33.2649, 14.6678) -> (33.2649, 13.5814)
  line L132 (33.2649, 13.5814) -> (31.9595, 12.593)
  line L133 (31.9595, 12.593) -> (31.9595, 12.2702)
  line L134 (31.9595, 12.2702) -> (33.2649, 12.2702)
  line L135 (33.2649, 12.2702) -> (33.2649, 11.3827)
  line L136 (33.2649, 11.3827) -> (29.7089, 11.3827)
  line L137 (29.7089, 11.3827) -> (29.7089, 12.812)
  spline S122 degree 2 poles (29.7089, 12.812) (29.7089, 13.1088) (29.7838, 13.5468) (29.8991, 13.7341) knots 0 0 0 1 2 2 2
  spline S123 degree 2 poles (29.8991, 13.7341) (30.0201, 13.9243) (30.3976, 14.1491) (30.6858, 14.1491) knots 0 0 0 1 2 2 2
  spline S124 degree 2 poles (30.6858, 14.1491) (31.0921, 14.1491) (31.6022, 13.7802) (31.752, 13.4719) knots 0 0 0 1 2 2 2
  line L138 (31.752, 13.4719) -> (33.2649, 14.6678)
  spline S125 degree 2 poles (30.7982, 13.2327) (30.6627, 13.2327) (30.4697, 13.129) (30.4178, 13.0108) knots 0 0 0 1 2 2 2
  spline S126 degree 2 poles (30.4178, 13.0108) (30.3832, 12.9272) (30.363, 12.7226) (30.363, 12.5699) knots 0 0 0 1 2 2 2
  line L139 (30.363, 12.5699) -> (30.363, 12.2702)
  line L140 (30.363, 12.2702) -> (31.3198, 12.2702)
  line L141 (31.3198, 12.2702) -> (31.3198, 12.5267)
  spline S127 degree 2 poles (31.3198, 12.5267) (31.3198, 12.7111) (31.2736, 12.9733) (31.2016, 13.0627) knots 0 0 0 1 2 2 2
  spline S128 degree 2 poles (31.2016, 13.0627) (31.1324, 13.1491) (30.948, 13.2327) (30.7982, 13.2327) knots 0 0 0 1 2 2 2
  spline S129 degree 2 poles (32.1756, 17.7742) (32.4407, 17.7742) (32.8413, 17.5725) (32.9738, 17.4054) knots 0 0 0 1 2 2 2
  spline S130 degree 2 poles (32.9738, 17.4054) (33.1323, 17.2037) (33.2649, 16.7253) (33.2649, 16.3536) knots 0 0 0 1 2 2 2
  line L142 (33.2649, 16.3536) -> (33.2649, 14.9329)
  line L143 (33.2649, 14.9329) -> (29.7089, 14.9329)
  line L144 (29.7089, 14.9329) -> (29.7089, 16.1864)
  spline S131 degree 2 poles (29.7089, 16.1864) (29.7089, 16.5783) (29.7694, 16.9818) (29.8645, 17.1576) knots 0 0 0 1 2 2 2
  spline S132 degree 2 poles (29.8645, 17.1576) (29.9654, 17.3506) (30.3112, 17.5379) (30.5359, 17.5379) knots 0 0 0 1 2 2 2
  spline S133 degree 2 poles (30.5359, 17.5379) (30.7953, 17.5379) (31.2016, 17.2786) (31.2967, 17.0481) knots 0 0 0 1 2 2 2
  line L145 (31.2967, 17.0481) -> (31.314, 17.0481)
  spline S134 degree 2 poles (31.314, 17.0481) (31.3832, 17.3794) (31.8125, 17.7742) (32.1756, 17.7742) knots 0 0 0 1 2 2 2
  spline S135 degree 2 poles (32.1612, 16.8521) (31.9941, 16.8521) (31.8068, 16.7195) (31.7578, 16.587) knots 0 0 0 1 2 2 2
  spline S136 degree 2 poles (31.7578, 16.587) (31.7261, 16.5063) (31.7203, 16.221) (31.7203, 15.9847) knots 0 0 0 1 2 2 2
  line L146 (31.7203, 15.9847) -> (31.7203, 15.8205)
  line L147 (31.7203, 15.8205) -> (32.6165, 15.8205)
  line L148 (32.6165, 15.8205) -> (32.6165, 15.8694)
  spline S137 degree 2 poles (32.6165, 15.8694) (32.6165, 16.2152) (32.6079, 16.4804) (32.5474, 16.6187) knots 0 0 0 1 2 2 2
  spline S138 degree 2 poles (32.5474, 16.6187) (32.4926, 16.7397) (32.2909, 16.8521) (32.1612, 16.8521) knots 0 0 0 1 2 2 2
  spline S139 degree 2 poles (30.7117, 16.6302) (30.6253, 16.6302) (30.4437, 16.5409) (30.4034, 16.4487) knots 0 0 0 1 2 2 2
  spline S140 degree 2 poles (30.4034, 16.4487) (30.363, 16.3622) (30.3573, 16.1202) (30.3573, 15.881) knots 0 0 0 1 2 2 2
  line L149 (30.3573, 15.881) -> (30.3573, 15.8205)
  line L150 (30.3573, 15.8205) -> (31.1123, 15.8205)
  line L151 (31.1123, 15.8205) -> (31.1123, 15.9328)
  spline S141 degree 2 poles (31.1123, 15.9328) (31.1123, 16.1605) (31.1036, 16.3449) (31.0575, 16.4429) knots 0 0 0 1 2 2 2
  spline S142 degree 2 poles (31.0575, 16.4429) (31.0056, 16.5495) (30.8299, 16.6302) (30.7117, 16.6302) knots 0 0 0 1 2 2 2
  spline S143 degree 2 poles (31.4869, 21.5233) (32.3514, 21.5233) (33.3398, 20.6012) (33.3398, 19.8001) knots 0 0 0 1 2 2 2
  spline S144 degree 2 poles (33.3398, 19.8001) (33.3398, 18.9961) (32.3399, 18.0797) (31.4869, 18.0797) knots 0 0 0 1 2 2 2
  spline S145 degree 2 poles (31.4869, 18.0797) (30.631, 18.0797) (29.634, 18.9961) (29.634, 19.8001) knots 0 0 0 1 2 2 2
  spline S146 degree 2 poles (29.634, 19.8001) (29.634, 20.6012) (30.6253, 21.5233) (31.4869, 21.5233) knots 0 0 0 1 2 2 2
  spline S147 degree 2 poles (31.4869, 20.6012) (31.167, 20.6012) (30.7204, 20.4715) (30.5792, 20.3591) knots 0 0 0 1 2 2 2
  spline S148 degree 2 poles (30.5792, 20.3591) (30.4322, 20.2467) (30.3054, 19.9586) (30.3054, 19.8029) knots 0 0 0 1 2 2 2
  spline S149 degree 2 poles (30.3054, 19.8029) (30.3054, 19.6387) (30.4235, 19.3707) (30.5734, 19.2468) knots 0 0 0 1 2 2 2
  spline S150 degree 2 poles (30.5734, 19.2468) (30.7117, 19.1373) (31.1699, 19.0018) (31.4869, 19.0018) knots 0 0 0 1 2 2 2
  spline S151 degree 2 poles (31.4869, 19.0018) (31.8154, 19.0018) (32.2477, 19.1315) (32.3946, 19.2439) knots 0 0 0 1 2 2 2
  spline S152 degree 2 poles (32.3946, 19.2439) (32.5416, 19.3563) (32.6684, 19.6473) (32.6684, 19.8029) knots 0 0 0 1 2 2 2
  spline S153 degree 2 poles (32.6684, 19.8029) (32.6684, 19.9614) (32.5329, 20.2554) (32.3889, 20.362) knots 0 0 0 1 2 2 2
  spline S154 degree 2 poles (32.3889, 20.362) (32.2332, 20.4773) (31.8212, 20.6012) (31.4869, 20.6012) knots 0 0 0 1 2 2 2
  line L152 (33.2649, 25.062) -> (33.2649, 24.0304)
  line L153 (33.2649, 24.0304) -> (32.1324, 23.3445)
  line L154 (32.1324, 23.3445) -> (33.2649, 22.6443)
  line L155 (33.2649, 22.6443) -> (33.2649, 21.6559)
  line L156 (33.2649, 21.6559) -> (31.4754, 22.8114)
  line L157 (31.4754, 22.8114) -> (29.7089, 21.702)
  line L158 (29.7089, 21.702) -> (29.7089, 22.7336)
  line L159 (29.7089, 22.7336) -> (30.7838, 23.3762)
  line L160 (30.7838, 23.3762) -> (29.7089, 24.0361)
  line L161 (29.7089, 24.0361) -> (29.7089, 25.0246)
  line L162 (29.7089, 25.0246) -> (31.4379, 23.9093)
  line L163 (31.4379, 23.9093) -> (33.2649, 25.062)
  point P0 (0, 0)
  point P1 (23.7791, 0)
  dimension "d4" = 20
  constraints: 1 horizontal alignment, 1 midpoint, 2 other
extrude "Extrusion8" cut sketch "Sketch7" against normal blind 1
body "Solid1"
